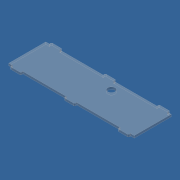
# Autodesk Inventor part: P1704_103
Saved by Autodesk Inventor 2015 (Build 190159000, 159)
## iProperties
Created: 2017-02-08
Part Number: P1704_103
Project: Manette
Material: Plastique PMMA
Description: Paroi avant - Chevalier
Document SubType Name: Modeling
Designer: Alexandre.PICOTTE
Authority: 176x58x3
Density: 1.188 g/cm^3
Appearance: Transparent - Clair
Mass: 33.2535 g
Surface Area: 202.588 cm^2
Volume: 27.9912 cm^3
Material number: ---
Author: Boris.GAUDARD
Autodesk Inventor part; units mm, degrees
ref_plane "Plan YZ" through (0, 0, 0) normal (1, 0, 0) x (0, 1, 0)
ref_plane "Plan XZ" through (0, 0, 0) normal (0, 1, 0) x (-1, 0, 0)
ref_plane "Plan XY" through (0, 0, 0) normal (0, 0, 1) x (1, 0, 0)
sketch "Esquisse12" plane through (0, 0, 0) normal (0, 0, 1) x (1, 0, 0)
  line L0 (-88, -26) -> (-88, 26)
  line L1 (-88, 26) -> (-83, 26)
  line L2 (-83, 26) -> (-83, 29)
  line L3 (-83, 29) -> (-68, 29)
  line L4 (-68, 29) -> (-68, 26)
  line L5 (7.5, 26) -> (7.5, 29)
  line L6 (7.5, 29) -> (-7.5, 29)
  line L7 (-7.5, 29) -> (-7.5, 26)
  line L8 (68, 26) -> (68, 29)
  line L9 (68, 29) -> (83, 29)
  line L10 (83, 29) -> (83, 26)
  line L11 (83, 26) -> (88, 26)
  line L12 (88, 26) -> (88, -26)
  line L13 (88, -26) -> (83, -26)
  line L14 (83, -26) -> (83, -29)
  line L15 (83, -29) -> (68, -29)
  line L16 (68, -29) -> (68, -26)
  line L17 (-7.5, -26) -> (-7.5, -29)
  line L18 (7.5, -29) -> (7.5, -26)
  line L19 (-68, -26) -> (-68, -29)
  line L20 (-83, -29) -> (-83, -26)
  line L21 (-88, -26) -> (-83, -26)
  line L22 (-83, -29) -> (-68, -29)
  line L23 (7.5, -29) -> (-7.5, -29)
  line L24 (-68, 26) -> (-7.5, 26)
  line L25 (7.5, 26) -> (68, 26)
  line L26 (7.5, -26) -> (68, -26)
  line L27 (-7.5, -26) -> (-68, -26)
  line L28 (-123.2, 0) -> (123.2, 0) construction
  line L29 (0, -40.6) -> (0, 40.6) construction
  point P0 (0, 0)
  dimension "d86" = 52
  dimension "d87" = 3
  dimension "d88" = 5
  dimension "d90" = 15
  dimension "d112" = 176
  constraints: 56 end point, 27 point on line, 10 perpendicular, 7 equal length, 3 collinear, 2 parallel, 2 vertical, 1 horizontal, 2 other
  measures "d86" distance of L0.start L0.end
  measures "d87" distance of L1.end L2.end
  measures "d88" distance of L0.end L1.end
  measures "d90" distance of L2.end L3.end
  measures "d112" distance between parallel lines of L12 L0
extrude "Extrusion5" add sketch "Esquisse12" along normal blind 3
sketch "Esquisse13" plane through (0, 0, 3) normal (0, 0, 1) x (1, 0, 0)
  point P0 (0, 0)
  point P1 (-83, 26)
  point P2 (-68, 26)
  point P3 (-83, -26)
  point P4 (-68, -26)
  point P5 (-7.5, -26)
  point P6 (7.5, -26)
  point P7 (68, -26)
  point P8 (83, -26)
  point P9 (83, 26)
  point P10 (68, 26)
  point P11 (-7.5, 26)
  point P12 (7.5, 26)
hole "Perçage6" at (-83, 26, 3) at (-68, 26, 3) at (-83, -26, 3) at (-68, -26, 3) at (-7.5, -26, 3) at (7.5, -26, 3) at (68, -26, 3) at (83, -26, 3) at (83, 26, 3) at (68, 26, 3) at (-7.5, 26, 3) at (7.5, 26, 3) direction (0, 0, -1) diameter 1 end through all
chamfer "Chanfrein3" distance 1 angle 45 12 edges at (-83, 29, 1.5) (-68, 29, 1.5) (-7.5, 29, 1.5) (7.5, 29, 1.5) (68, 29, 1.5) (83, 29, 1.5) (-83, -29, 1.5) (-68, -29, 1.5) (-7.5, -29, 1.5) (7.5, -29, 1.5) (68, -29, 1.5) (83, -29, 1.5)
sketch "Esquisse14" plane through (0, 0, 3) normal (0, 0, 1) x (1, 0, 0)
  circle A0 centre (16.2, 13.8) radius 5
  line L0 (-88, -26) -> (-88, 26) projected
  line L1 (67.5, -26) -> (8, -26) projected
  line L2 (88, 26) -> (88, -26) projected
  point P0 (0, 0)
  dimension "d108" = 39.8
  dimension "d109" = 10
  dimension "d113" = 71.8
  constraints: 1 centre point
  measures "d108" distance from line of L1 A0.centre
  measures "d109" diameter of A0
  measures "d113" distance from line of A0.centre L2
extrude "Extrusion6" cut sketch "Esquisse14" against normal through all
